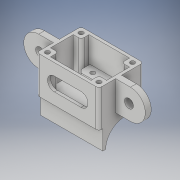
# Autodesk Inventor part: Caixa
Saved by Autodesk Inventor 2019 (Build 230136000, 136)
## iProperties
Created: 2021-05-27
Part Number: Caixa
Material: Generic
Document SubType Name: Modeling
Designer: hoope
Density: 1 g/cm^3
Appearance: Default
Author: hoope
Autodesk Inventor part; units mm, degrees
ref_plane "YZ Plane" through (0, 0, 0) normal (1, 0, 0) x (0, 1, 0)
ref_plane "XZ Plane" through (0, 0, 0) normal (0, 1, 0) x (-1, 0, 0)
ref_plane "XY Plane" through (0, 0, 0) normal (0, 0, 1) x (1, 0, 0)
sketch "Esboço1" plane through (0, 0, 0) normal (0, 1, 0) x (-1, 0, 0)
  line L0 (0, 0) -> (42, 0)
  line L1 (42, 0) -> (42, 30)
  line L2 (42, 30) -> (0, 30)
  line L3 (0, 30) -> (0, 0)
  dimension "d0" = 42
  dimension "d1" = 30
  constraints: 8 end point, 2 parallel, 1 horizontal, 1 perpendicular
  measures "d0" distance of L2.end L1.end
  measures "d1" distance of L1.end L0.end
extrude "Extrusão1" add sketch "Esboço1" along normal blind 25
shell "Casca1" thickness 2 removed faces 1 at (-14, 25, 20)
sketch "Esboço2" plane through (-42, 0, 30) normal (0, 0, 1) x (1, 0, 0)
  arc A0 (12, 17.15) -> (12, 7.85) centre (12, 12.5) ccw
  line L0 (0, 25) -> (42, 25) projected
  arc A1 (30, 7.85) -> (30, 17.15) centre (30, 12.5) ccw
  line L1 (42, 0) -> (42, 25) projected
  line L2 (12, 17.15) -> (30, 17.15)
  line L3 (30, 7.85) -> (12, 7.85)
  dimension "d5" = 9.3
  dimension "d6" = 12.5
  dimension "d7" = 9.3
  dimension "d8" = 18
  dimension "d9" = 12
  constraints: 4 end point, 4 point on circle, 2 centre point, 1 horizontal, 1 parallel
  measures "d5" diameter of A0
  measures "d6" distance from line of L0 A0.centre
  measures "d7" diameter of A1
  measures "d8" distance of A1.centre A0.centre
  measures "d9" distance from line of L1 A1.centre
extrude "Extrusão2" cut sketch "Esboço2" against normal blind 10
sketch "Esboço3" plane through (-40, 2, 2) normal (0, 1, 0) x (1, 0, 0)
  line L0 (38, 0) -> (0, 0) projected
  line L1 (0, 0) -> (5.3, 0)
  line L2 (5.3, 0) -> (5.3, -5.3)
  line L3 (5.3, -5.3) -> (0, -5.3)
  line L4 (0, -5.3) -> (0, 0)
  line L5 (38, 0) -> (32.7, 0)
  line L6 (32.7, 0) -> (32.7, -5.3)
  line L7 (32.7, -5.3) -> (38, -5.3)
  line L8 (38, -5.3) -> (38, 0)
  line L9 (38, -26) -> (32.7, -26)
  line L10 (32.7, -26) -> (32.7, -20.7)
  line L11 (32.7, -20.7) -> (38, -20.7)
  line L12 (38, -20.7) -> (38, -26)
  line L13 (38, -26) -> (0, -26) projected
  line L14 (0, -26) -> (5.3, -26)
  line L15 (5.3, -26) -> (5.3, -20.7)
  line L16 (5.3, -20.7) -> (0, -20.7)
  line L17 (0, -20.7) -> (0, -26)
  point P0 (40, 2)
  dimension "d12" = 5.3
  dimension "d13" = 5.3
  dimension "d14" = 5.3
  dimension "d15" = 5.3
  dimension "d16" = 5.3
  dimension "d17" = 5.3
  dimension "d18" = 5.3
  dimension "d19" = 5.3
  constraints: 32 end point, 8 parallel, 4 horizontal, 4 perpendicular
  measures "d12" distance of L2.end L3.end
  measures "d13" distance of L1.end L2.end
  measures "d14" distance of L7.end L6.end
  measures "d15" distance of L6.end L5.end
  measures "d16" distance of L10.end L11.end
  measures "d17" distance of L9.end L10.end
  measures "d18" distance of L16.end L15.end
  measures "d19" distance of L15.end L14.end
extrude "Extrusão3" add sketch "Esboço3" along normal blind 23
sketch "Esboço4" plane through (-34.7, 2, 2) normal (0, 1, 0) x (1, 0, 0)
  line L0 (27.4, 0) -> (27.4, -5.3) projected
  line L1 (0, -5.3) -> (0, 0) projected
  line L2 (0, 0) -> (27.4, 0) projected
  line L3 (27.4, 0) -> (0, 0) projected
  line L4 (0.7, 0) -> (26.7, 0)
  line L5 (26.7, 0) -> (26.7, -8)
  line L6 (26.7, -8) -> (0.7, -8)
  line L7 (0.7, -8) -> (0.7, 0)
  line L8 (19.0046, -4) -> (20.5923, -1.25)
  line L9 (23.7677, -6.75) -> (25.3554, -4)
  line L10 (20.5923, -1.25) -> (23.7677, -1.25)
  line L11 (20.5923, -6.75) -> (23.7677, -6.75)
  line L12 (19.0046, -4) -> (20.5923, -6.75)
  line L13 (23.7677, -1.25) -> (25.3554, -4)
  line L14 (3.4446, -4) -> (5.0323, -1.25)
  line L15 (5.0323, -6.75) -> (8.2077, -6.75)
  line L16 (3.4446, -4) -> (5.0323, -6.75)
  line L17 (5.0323, -1.25) -> (8.2077, -1.25)
  line L18 (20.5923, -1.25) -> (23.7677, -1.25)
  line L19 (8.2077, -1.25) -> (9.7954, -4)
  line L20 (8.2077, -6.75) -> (9.7954, -4)
  point P0 (34.7, 2)
  dimension "d33" = 26
  dimension "d34" = 8
  dimension "d35" = 0.7
  dimension "d208" = 5.5
  dimension "d210" = 5.5
  dimension "d213" = 120
  dimension "d214" = 120
  dimension "d223" = 120
  dimension "d225" = 120
  dimension "d227" = 120
  constraints: 34 end point, 6 horizontal, 3 parallel, 1 perpendicular, 1 point on line
  measures "d33" distance between parallel lines of L5 L7
  measures "d34" distance between parallel lines of L4 L6
  measures "d35" distance between parallel lines of L0 L5
  measures "d208" distance between parallel lines of L9 L8
  measures "d210" distance between parallel lines of L11 L10
  measures "d213" angle of L8 L10
  measures "d214" angle of L8 L12
  measures "d223" angle of L14 L16
  measures "d225" angle of L19 L17
  measures "d227" angle of L19 L20
sketch "Esboço6" plane through (0, 25, 0) normal (0, 1, 0) x (1, 0, 0)
  circle A0 centre (-38.35, -3.65) radius 1.505
  line L0 (0, 0) -> (-42, 0) projected
  line L1 (-42, 0) -> (-42, -30) projected
  circle A1 centre (-3.65, -26.35) radius 1.505
  line L2 (0, -30) -> (0, 0) projected
  line L3 (-42, -30) -> (0, -30) projected
  circle A2 centre (-3.65, -3.65) radius 1.505
  circle A3 centre (-38.35, -26.35) radius 1.505
  dimension "d48" = 3.01
  dimension "d49" = 3.65
  dimension "d50" = 3.65
  dimension "d51" = 3.01
  dimension "d52" = 3.65
  dimension "d53" = 3.65
  dimension "d54" = 3.01
  dimension "d55" = 3.01
  dimension "d56" = 3.65
  dimension "d57" = 3.65
  dimension "d65" = 3.65
  dimension "d66" = 3.65
  constraints: 4 centre point
  measures "d48" diameter of A0
  measures "d49" distance from line of L0 A0.centre
  measures "d50" distance from line of L1 A0.centre
  measures "d51" diameter of A1
  measures "d52" distance from line of L2 A1.centre
  measures "d53" distance from line of L3 A1.centre
  measures "d54" diameter of A2
  measures "d55" diameter of A3
  measures "d56" distance from line of L1 A3.centre
  measures "d57" distance from line of L3 A3.centre
  measures "d65" distance from line of L0 A2.centre
  measures "d66" distance from line of L2 A2.centre
extrude "Extrusão6" cut sketch "Esboço6" against normal blind 15 contours A0 | A1 | A2 | A3
fillet "Arredondamento1" radius 2 4 edges at (-42, 12.5, 30) (0, 12.5, 30) (0, 12.5, 0) (-42, 12.5, 0)
fillet "Arredondamento2" radius 2 4 edges at (-34.7, 13.5, 7.3) (-7.3, 13.5, 7.3) (-34.7, 13.5, 22.7) (-7.3, 13.5, 22.7)
sketch "Esboço40" plane through (-42, 0, 2) normal (-1, 0, 0) x (0, 0, 1)
  arc A0 (23.4, -13) -> (0, -6.1589) centre (10.7, -13) ccw
  line L0 (0, 0) -> (26, 0) projected
  line L1 (-2, 25) -> (-2, 0) projected
  line L2 (0, 0) -> (0, 25) projected
  line L3 (-2, 0) -> (-2, -6.1589)
  line L4 (-2, -6.1589) -> (0, -6.1589)
  line L5 (25.4, -13) -> (25.4, 0)
  line L6 (26, 25) -> (26, 0) projected
  line L7 (23.4, -13) -> (25.4, -13)
  line L8 (0, 0) -> (-2, 0) projected
  line L9 (25.4, 0) -> (-2, 0)
  dimension "d184" = 25.4
  dimension "d185" = 13
  dimension "d186" = 12.7
  dimension "d187" = 14.7
  constraints: 10 end point, 2 perpendicular, 2 point on circle, 1 centre point, 1 horizontal, 1 parallel, 1 point on line, 1 vertical
  measures "d184" diameter of A0
  measures "d185" distance from line of L0 A0.centre
  measures "d186" distance from line of L1 A0.centre
  measures "d187" distance from line of L5 A0.centre
extrude "Extrusão30" add sketch "Esboço40" against normal blind 42
fillet "Arredondamento10" radius 2 2 edges at (-42, -3.0795, 0) (0, -3.0795, 0)
sketch "Esboço41" plane through (0, 0, 28) normal (1, 0, 0) x (0, 0, -1)
  line L0 (9.3, 25) -> (13.3, 25)
  line L1 (13.3, 25) -> (13.3, 5)
  line L2 (13.3, 5) -> (9.3, 5)
  line L3 (9.3, 5) -> (9.3, 25)
  line L4 (26, 25) -> (26, -6.1589) projected
  line L5 (0, 25) -> (26, 25) projected
  point P0 (28, 0)
  dimension "d191" = 4
  dimension "d192" = 20
  dimension "d193" = 12.7
  constraints: 8 end point, 2 parallel, 1 horizontal, 1 perpendicular
  measures "d191" distance of L1.end L2.end
  measures "d192" distance of L0.end L1.end
  measures "d193" distance between parallel lines of L4 L1
extrude "Extrusão31" add sketch "Esboço41" along normal blind 20
sketch "Esboço42" plane through (-42, 0, 28) normal (-1, 0, 0) x (0, 0, 1)
  line L0 (-9.3, 5) -> (-9.3, 25) projected
  line L1 (-13.3, 25) -> (-13.3, 5) projected
  line L2 (-9.3, 25) -> (-13.3, 25)
  line L3 (-13.3, 25) -> (-13.3, 5)
  line L4 (-13.3, 5) -> (-9.3, 5)
  line L5 (-9.3, 5) -> (-9.3, 25)
  point P0 (-28, 0)
  constraints: 8 end point, 2 parallel, 1 horizontal, 1 perpendicular
extrude "Extrusão32" add sketch "Esboço42" along normal blind 20
fillet "Arredondamento11" radius 10 4 edges at (-62, 25, 16.7) (-62, 5, 16.7) (20, 25, 16.7) (20, 5, 16.7)
sketch "Esboço44" plane through (-42, 5, 18.7) normal (0, 0, 1) x (1, 0, 0)
  circle A0 centre (51, 10) radius 3
  circle A1 centre (-9, 10) radius 3
  line L0 (0, 20) -> (0, -5) projected
  line L1 (42, -5) -> (42, 20) projected
  dimension "d202" = 6
  dimension "d203" = 6
  dimension "d204" = 9
  dimension "d205" = 9
  constraints: 2 centre point
  measures "d202" diameter of A0
  measures "d203" diameter of A1
  measures "d204" distance from line of L0 A1.centre
  measures "d205" distance from line of L1 A0.centre
extrude "Extrusão33" cut sketch "Esboço44" against normal blind 20
extrude "Extrusão34" add sketch "Esboço4" along normal blind 3
sketch "Esboço47" plane through (-34.7, 5, 2) normal (0, 1, 0) x (1, 0, 0)
  line L0 (0.7, -8) -> (0.7, 0) projected
  line L1 (0.7, -8) -> (26.7, -8)
  line L2 (26.7, -8) -> (26.7, 0)
  line L3 (26.7, 0) -> (0.7, 0)
  line L4 (0.7, 0) -> (0.7, -8)
  line L5 (26.7, -8) -> (26.7, 0) projected
  point P0 (34.7, 2)
  dimension "d239" = 0
  constraints: 8 end point, 2 parallel, 1 horizontal, 1 perpendicular
  measures "d239" distance between parallel lines of L5 L2
extrude "Extrusão35" add sketch "Esboço47" along normal blind 3
sketch "Esboço48" plane through (-34.7, 8, 2) normal (0, 1, 0) x (1, 0, 0)
  circle A0 centre (6.62, -4) radius 1.5
  circle A1 centre (22.18, -4) radius 1.5
  point P0 (34.7, 2)
  dimension "d232" = 3
  dimension "d233" = 3
  constraints: 2 centre point
  measures "d232" diameter of A0
  measures "d233" diameter of A1
extrude "Extrusão36" cut sketch "Esboço48" against normal blind 3
chamfer "Chanfro4" distance 2 angle 45 2 edges at (-34, 5, 10) (-8, 5, 10)
